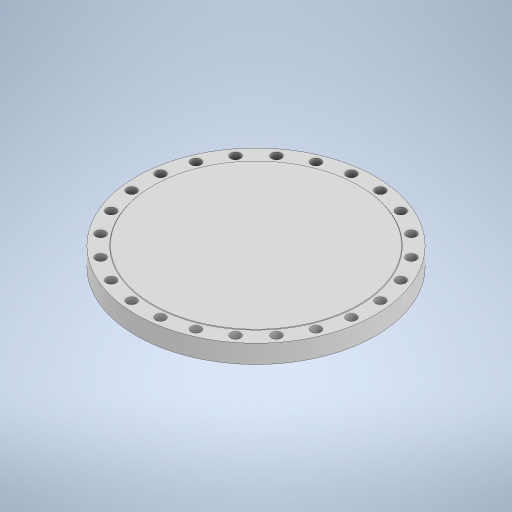
# Autodesk Inventor part: ASME-A150-26B
Saved by Autodesk Inventor 2023 (Build 270158000, 158)
## iProperties
Created: 2023-11-03
Part Number: ASME-A150-26B
Material: Generic
Document SubType Name: Modeling
Designer: Admin
Density: 1 g/cm^3
Appearance: Default
Author: Admin
Autodesk Inventor part; units mm, degrees
ref_plane "YZ Plane" through (0, 0, 0) normal (1, 0, 0) x (0, 1, 0)
ref_plane "XZ Plane" through (0, 0, 0) normal (0, 1, 0) x (-1, 0, 0)
ref_plane "XY Plane" through (0, 0, 0) normal (0, 0, 1) x (1, 0, 0)
sketch "Sketch1" plane through (0, 0, 0) normal (0, 0, 1) x (1, 0, 0)
  line L0 (0, 0) -> (0, 68.3895)
  line L1 (-11.176, 0) -> (-17.526, 0)
  line L2 (0, 0) -> (-434.975, 0)
  line L3 (-434.975, 0) -> (-434.975, 66.802)
  line L4 (-434.975, 66.802) -> (-376.2375, 66.802)
  line L5 (-403.225, 66.802) -> (-403.225, 0) construction
  line L6 (0, 68.3895) -> (-374.65, 68.3895)
  line L7 (-376.2375, 66.802) -> (-374.65, 68.3895)
  dimension "Thickness" = 66.802
  dimension "OD" = 869.95
  dimension "BC" = 806.45
  dimension "d25" = 1.5875
  dimension "d26" = 135
  dimension "R" = 749.3
  constraints: 16 end point, 4 horizontal, 3 vertical, 2 point on line, 1 horizontal alignment
  measures "Thickness" distance of L2.end L3.end
  measures "OD" diameter of L3 L0
  measures "BC" diameter of L5 L0
  measures "d25" distance between parallel lines of L4 L6
  measures "d26" angle of L6 L7
  measures "R" diameter of L6.end L0
revolve "Revolution1" add sketch "Sketch1" angle 360 about axis through (0, 0, 0) along (0, 1, 0)
sketch "Sketch2" plane through (0, 66.802, 0) normal (0, 1, 0) x (1, 0, 0)
  line L0 (0, 0) -> (0, 434.975) construction
  circle A0 centre (0, 0) radius 434.975 projected
  line L1 (0, 0) -> (52.6314, 399.7754) construction
  dimension "d11" = 7.5
  dimension "d12" = 403.225
  constraints: 4 end point, 1 coincident, 1 vertical, 1 vertical alignment, 1 other
  measures "d11" angle of L1 L0
  measures "d12" distance of L1.start L1.end
hole "Hole1" at (52.6314, 66.802, -399.7754) direction (0, -1, 0) diameter 34.925 depth 66.802
pattern_circular "Circular Pattern1" count 24 over 360 about axis through (0, -10, 0) along (0, 1, 0) of "Hole1"
equation "\"d12\" = 0.5 * BC"
body "Solid1"
